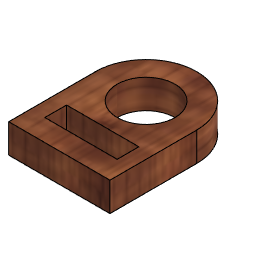
Practice1 (Autodesk Fusion 360 design; units mm, degrees)
Autodesk Fusion 360 part; units mm, degrees
sketch "Sketch1" plane through (0, 0, 0) normal (0, 0, 1) x (1, 0, 0)
  line L0 (0, 0) -> (70, 0)
  line L1 (70, 0) -> (70, 60)
  line L2 (0, 60) -> (0, 0)
  circle A0 centre (35, 60) radius 20
  line L3 (10, 15) -> (60, 15)
  line L4 (10, 30) -> (60, 30)
  line L5 (10, 30) -> (10, 15)
  line L6 (60, 30) -> (60, 15)
  arc A1 (70, 60) -> (0, 60) centre (35, 60) ccw
  dimension "d1" = 70
  dimension "d2" = 60
  dimension "d14" = 10
  dimension "d15" = 15
  dimension "d17" = 40
  dimension "d18" = 35
  dimension "d20" = 50
  dimension "d21" = 15
  constraint horizontal L0
  constraint vertical L1
  constraint vertical L2
  constraint coincident L0.start L2.end
  constraint concentric A0 A1
  constraint perpendicular L2 L3
  constraint perpendicular L3 L5
  constraint tangent L1 A1
  constraint horizontal L4
  constraint vertical L6
  measures "d1" distance of L0.start L0.end
  measures "d2" distance of L0.start L2.start
  measures "d14" distance of L2 L5
  measures "d15" distance of L0 L3
  measures "d17" diameter of A0
  measures "d18" radius of A1
  measures "d20" distance of L4.start L4.end
  measures "d21" distance of L3.end L4.end
extrude "Extrude1" add sketch "Sketch1" along normal mid plane 20
